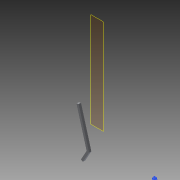
# Autodesk Inventor part: V-Arm
Saved by Autodesk Inventor 2013 (Build 170138000, 138)
## iProperties
Created: 2014-01-16
Part Number: V-Arm
Material: Generic
Document SubType Name: Modeling
Designer: 215152
Density: 1 g/cm^3
Author: 215152
Autodesk Inventor part; units mm, degrees
ref_plane "YZ Plane" through (0, 0, 0) normal (1, 0, 0) x (0, 1, 0)
ref_plane "XZ Plane" through (0, 0, 0) normal (0, 1, 0) x (-1, 0, 0)
ref_plane "XY Plane" through (0, 0, 0) normal (0, 0, 1) x (1, 0, 0)
ref_plane "Work Plane1" through (-0.0049, -0.13, 0) normal (0, 0, 1) x (1, 0, 0)
sketch "Sketch1" plane through (-0.0049, -0.13, 0) normal (0, 0, 1) x (1, 0, 0)
  line L0 (0.0049, 0.13) -> (-63.4951, 0.13)
  line L1 (-63.4951, 0.13) -> (-63.4951, -482.47)
  line L2 (-63.4951, -482.47) -> (0.0049, -482.47)
  line L3 (0.0049, -482.47) -> (0.0049, 0.13)
  line L4 (-63.4951, -482.47) -> (114.3049, -482.47)
  line L5 (-63.4951, -482.47) -> (114.3049, -482.47) construction
  line L6 (-63.4951, -482.47) -> (63.5049, -482.47)
  line L7 (63.5049, -482.47) -> (63.5049, -406.27)
  line L8 (63.5049, -406.27) -> (-63.4951, -406.27)
  line L9 (-63.4951, -406.27) -> (-63.4951, -482.47)
  line L10 (-63.4951, -482.47) -> (-63.4951, -914.27)
  line L11 (-63.4951, -482.47) -> (368.3049, -482.47) construction
  line L12 (-63.4951, -914.27) -> (114.3049, -914.27)
  line L13 (114.3049, -914.27) -> (114.3049, -482.47)
  line L14 (-63.4951, -406.27) -> (-63.4951, -393.57)
  line L15 (-63.4951, -406.27) -> (-50.7951, -406.27) construction
  line L16 (-63.4951, -393.57) -> (-317.4951, -393.57)
  line L17 (-63.4951, -393.57) -> (190.5049, -393.57) construction
  line L18 (-63.4951, -393.57) -> (-317.4951, -393.57)
  line L19 (-317.4951, -393.57) -> (-317.4951, -914.27)
  line L20 (-317.4951, -914.27) -> (-63.4951, -914.27)
  line L21 (-63.4951, -914.27) -> (-63.4951, -393.57)
  line L22 (-63.4951, -393.57) -> (-177.7951, -393.57)
  line L23 (-177.7951, -393.57) -> (114.3049, -685.67)
  line L24 (114.3049, -685.67) -> (114.3049, -914.27)
  line L25 (-177.7951, -393.57) -> (114.3049, -685.6537)
  line L26 (-177.7951, -393.57) -> (-177.7951, -990.597)
  line L27 (-177.7951, -393.57) -> (419.2319, -393.57) construction
  line L28 (-177.7951, -990.597) -> (-65.9571, -791.2225)
  line L29 (-177.7951, -990.597) -> (50.8049, -990.597) construction
  line L30 (-65.9571, -791.2225) -> (-177.7951, -393.57)
  line L31 (-134.9799, -914.27) -> (-157.1327, -901.8436)
  line L32 (-134.9799, -914.27) -> (-109.5799, -914.27) construction
  line L33 (-157.1327, -901.8436) -> (-95.0804, -791.2225)
  line L34 (-75.3464, -757.8376) -> (-99.7978, -764.7145)
  line L35 (-95.0804, -791.2225) -> (-93.2568, -787.9716)
  line L36 (-93.2568, -787.9716) -> (-204.1924, -393.57)
  line L37 (-93.2568, -787.9716) -> (316.4496, -787.9716) construction
  line L38 (-190.4951, -393.57) -> (-193.9339, -381.3444)
  line L39 (-190.4951, -393.57) -> (-177.7951, -393.57) construction
  line L40 (-204.1924, -393.57) -> (-207.1501, -383.0548)
  line L41 (-193.9339, -381.3444) -> (-206.6269, -384.9147)
  line L42 (-206.6269, -384.9147) -> (-176.4218, -376.4187)
  line L43 (-177.7951, -393.57) -> (-182.165, -378.0341)
  line L44 (-182.165, -378.0341) -> (-206.6269, -384.9147)
  line L45 (-206.6269, -384.9147) -> (-93.2568, -787.9716)
  line L46 (-190.4951, -393.57) -> (-177.7951, -393.57)
  line L47 (-177.7951, -393.57) -> (-182.165, -378.0341)
  line L48 (-182.165, -378.0341) -> (-193.9339, -381.3444)
  line L49 (-193.9339, -381.3444) -> (-190.4951, -393.57)
  dimension "d0" = 63.5
  dimension "d1" = 482.6
  dimension "d2" = 177.8
  dimension "d3" = 0
  dimension "d4" = 127
  dimension "d5" = 76.2
  dimension "d6" = 431.8
  dimension "d7" = 90
  dimension "d8" = 12.7
  dimension "d9" = 90
  dimension "d10" = 254
  dimension "d11" = 180
  dimension "d12" = 254
  dimension "d13" = 520.7
  dimension "d14" = 114.3
  dimension "d15" = 45
  dimension "d16" = 413.0802
  dimension "d17" = 597.027
  dimension "d18" = 90
  dimension "d19" = 228.6
  dimension "d20" = 60.71
  dimension "d21" = 25.4
  dimension "d22" = 150.71
  dimension "d23" = 25.4
  dimension "d25" = 105.71
  dimension "d26" = 12.7
  dimension "d27" = 105.71
  constraints: 100 end point, 12 horizontal, 12 parallel, 11 perpendicular, 9 collinear, 9 equal length, 9 point on line, 1 midpoint
  measures "d0" distance of L2.end L1.end
  measures "d1" distance of L1.end L0.end
  measures "d2" distance of L1.end L4.end
  measures "d3" distance between parallel lines of L4 L5
  measures "d4" distance of L8.end L7.end
  measures "d5" distance of L7.end L6.end
  measures "d6" distance of L1.end L10.end
  measures "d7" angle of L10 L11
  measures "d8" distance of L8.end L14.end
  measures "d9" angle of L15 L14
  measures "d10" distance of L14.end L16.end
  measures "d11" angle of L16 L17
  measures "d12" distance of L20.end L19.end
  measures "d13" distance of L19.end L18.end
  measures "d14" distance of L14.end L22.end
  measures "d15" angle of L23 L22
  measures "d16" distance of L22.end L25.end
  measures "d17" distance of L22.end L26.end
  measures "d18" angle of L26 L27
  measures "d19" distance of L26.end L28.end
  measures "d20" angle of L29 L28
  measures "d21" distance of L31.start L31.end
  measures "d22" angle of L32 L31
  measures "d23" distance of L34.start L34.end
  measures "d25" angle of L37 L36
  measures "d26" distance of L38.start L38.end
  measures "d27" angle of L39 L38
extrude "Extrusion1" add sketch "Sketch1" along normal blind 25.4 contours L26 L36 L16 | L30 L34 L36 L26 | L16 L38 L42 L43 | L16 L40 L41 L38 | L30 L28 L31 L33 L35 L36 L34
sketch "Sketch2" plane through (-0.0049, -0.13, 25.4) normal (0, 0, 1) x (1, 0, 0)
  line L0 (-182.165, -378.0341) -> (-206.6269, -384.9147) projected
  line L1 (-206.6269, -384.9147) -> (-182.165, -378.0341)
  line L2 (-182.165, -378.0341) -> (-194.396, -381.4744)
  line L3 (-194.396, -381.4744) -> (-190.9572, -393.7)
  circle A0 centre (-190.9572, -393.7) radius 3.175
  point P0 (0.0049, 0.13)
  dimension "d30" = 12.7
  dimension "d31" = 6.35
  constraints: 6 end point, 1 centre point, 1 coincident, 1 collinear, 1 midpoint, 1 perpendicular
  measures "d30" distance of L2.end L3.end
  measures "d31" diameter of A0
extrude "Extrusion2" cut sketch "Sketch2" against normal blind 25.4
body "Solid1"
